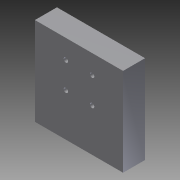
# Autodesk Inventor part: mixer mount
Saved by Autodesk Inventor 2011 (Build 150239000, 239)
## iProperties
Created: 2014-04-04
Part Number: mixer mount
Document SubType Name: Modeling
Designer: Devon
Density: 1 g/cm^3
Author: Devon
Autodesk Inventor part; units mm, degrees
ref_plane "YZ Plane" through (0, 0, 0) normal (1, 0, 0) x (0, 1, 0)
ref_plane "XZ Plane" through (0, 0, 0) normal (0, 1, 0) x (-1, 0, 0)
ref_plane "XY Plane" through (0, 0, 0) normal (0, 0, 1) x (1, 0, 0)
sketch "Sketch1" plane through (0, 0, 0) normal (0, 0, 1) x (1, 0, 0)
  line L0 (-23.6409, 18.7983) -> (77.9591, 18.7983)
  line L1 (77.9591, 18.7983) -> (77.9591, -82.8017)
  line L2 (77.9591, -82.8017) -> (-23.6409, -82.8017)
  line L3 (-23.6409, -82.8017) -> (-23.6409, 18.7983)
  point P0 (0, 0)
  dimension "d0" = 101.6
  dimension "d1" = 101.6
  constraints: 8 end point, 2 parallel, 1 horizontal, 1 perpendicular
  measures "d0" distance of L1.end L2.end
  measures "d1" distance of L0.end L1.end
extrude "Extrusion1" add sketch "Sketch1" along normal blind 25.4
sketch "Sketch2" plane through (0, 0, 25.4) normal (0, 0, 1) x (1, 0, 0)
  line L0 (-23.6409, 18.7983) -> (77.9591, 18.7983) projected
  line L1 (27.1591, 18.7983) -> (52.8131, 18.7983)
  line L2 (27.1591, 18.7983) -> (1.5051, 18.7983)
  line L3 (1.5051, 18.7983) -> (12.0461, 18.7983)
  line L4 (52.8131, 18.7983) -> (42.2721, 18.7983)
  line L5 (12.0461, 18.7983) -> (12.0461, -3.4267)
  line L6 (12.0461, 18.7983) -> (12.0461, -33.5257)
  line L7 (42.2721, 18.7983) -> (42.2721, -3.4267)
  line L8 (42.2721, -3.4267) -> (42.2721, -33.5257)
  point P0 (0, 0)
  dimension "d4" = 25.654
  dimension "d5" = 25.654
  dimension "d6" = 10.541
  dimension "d7" = 10.541
  dimension "d8" = 22.225
  dimension "d9" = 52.324
  constraints: 16 end point, 4 point on line, 2 collinear, 1 midpoint, 1 parallel, 1 perpendicular
  measures "d4" distance of L1.start L1.end
  measures "d5" distance of L1.start L2.end
  measures "d6" distance of L2.end L3.end
  measures "d7" distance of L1.end L4.end
  measures "d8" distance of L3.end L5.end
  measures "d9" distance of L3.end L6.end
hole "Hole1" at (12.0461, -3.4267, 25.4) at (42.2721, -3.4267, 25.4) at (42.2721, -33.5257, 25.4) at (12.0461, -33.5257, 25.4) direction (0, 0, -1) diameter 5.1054 depth 25.4 tip angle 118 clearance for "Socket Head Cap Screw" size "#10" standard "Ansi Unified Screw Threads"
sketch "Sketch3" plane through (-23.6409, -82.8017, 0) normal (0, -1, 0) x (1, 0, 0)
  line L0 (101.6, 25.4) -> (0, 25.4) projected
  line L1 (101.6, 0) -> (0, 0) projected
  line L2 (50.8, 25.4) -> (50.8, 0)
  line L3 (50.8, 12.7) -> (56.2489, 12.7)
  point P0 (23.6409, 0)
  constraints: 4 end point, 3 midpoint, 1 perpendicular
hole "Hole2" at (27.1591, -82.8017, 12.7) direction (0, 1, 0) diameter 4.9784 depth 12.7 tip angle 118 thread size "1/4-20 UNC" class "2B" standard "ANSI Unified Screw Threads"
body "Solid1"
